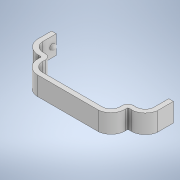
# Autodesk Inventor part: NEMA23_Shroud_Cover
Saved by Autodesk Inventor 2021 (Build 250183000, 183)
## iProperties
Created: 2021-04-01
Part Number: NEMA23_Shroud_Cover
Material: Generic
Document SubType Name: Modeling
Designer: Jorian Brusind
Density: 1 g/cm^3
Appearance: Default
Author: Jorian Brusind
Autodesk Inventor part; units mm, degrees
ref_plane "YZ Plane" through (0, 0, 0) normal (1, 0, 0) x (0, 1, 0)
ref_plane "XZ Plane" through (0, 0, 0) normal (0, 1, 0) x (-1, 0, 0)
ref_plane "XY Plane" through (0, 0, 0) normal (0, 0, 1) x (1, 0, 0)
sketch "Sketch1" plane through (0, 0, 0) normal (0, 1, 0) x (-1, 0, 0)
  arc A0 (-51.5269, -6.9638) -> (-48.7189, -4.3924) centre (-51.6928, -3.9638) ccw
  line L0 (-51.5269, -6.9638) -> (-53.0277, -6.9638)
  arc A1 (-53.0277, -6.9638) -> (-55.8647, -7.8466) centre (-53.0278, -11.9638) ccw
  arc A2 (-48.0059, -0.3912) -> (-48.7189, -2.9645) centre (-43.7189, -2.9645) ccw
  line L1 (-48.7189, -2.9645) -> (-48.7189, -4.3924)
  arc A3 (-44.3192, 1.9993) -> (-48.0059, -0.3912) centre (-43.7189, -2.9645) ccw
  arc A4 (-55.8647, -7.8466) -> (-57.9428, -11.046) centre (-53.0278, -11.9639) ccw
  arc A5 (-7.9592, -0.1638) -> (-12.0937, 1.9993) centre (-12.0765, -3.0006) ccw
  arc A6 (-7.0769, -2.9368) -> (-7.9592, -0.1638) centre (-12.0765, -3.0006) ccw
  arc A7 (-7.0717, -4.4481) -> (-4.4894, -7.4079) centre (-4.0718, -4.4371) ccw
  line L2 (-7.0717, -4.4481) -> (-7.0769, -2.9368)
  arc A8 (-0.4247, -8.1232) -> (-3.0701, -7.403) centre (-3.0107, -12.4029) ccw
  line L3 (-3.0701, -7.403) -> (-4.4894, -7.4079)
  arc A9 (2.1302, -12.0566) -> (-0.4247, -8.1232) centre (-2.8554, -12.4986) ccw
  line L4 (2.1302, -12.0566) -> (2.1302, -17.0566)
  line L5 (-57.9428, -11.046) -> (-57.9439, -17.046)
  line L6 (-57.9439, -17.046) -> (2.1302, -17.0566)
  line L7 (-44.3192, 1.9993) -> (-12.0937, 1.9993)
  arc A10 (-6.0769, -2.9289) -> (-7.1357, 0.4036) centre (-12.0765, -3.0006) ccw
  arc A11 (-7.1357, 0.4036) -> (-12.0953, 2.9993) centre (-12.0765, -3.0006) ccw
  line L8 (-12.0953, 2.9993) -> (-44.3767, 2.9993)
  arc A12 (-44.3767, 2.9993) -> (-48.8633, 0.1235) centre (-43.7189, -2.9645) ccw
  arc A13 (-48.8633, 0.1235) -> (-49.7189, -2.9645) centre (-43.7189, -2.9645) ccw
  line L9 (-49.7189, -2.9645) -> (-49.7189, -4.3135)
  arc A14 (-51.5573, -5.9638) -> (-49.7189, -4.3135) centre (-51.6928, -3.9638) ccw
  line L10 (-51.5573, -5.9638) -> (-53.0277, -5.9638)
  arc A15 (-53.0277, -5.9638) -> (-56.4321, -7.0231) centre (-53.0278, -11.9638) ccw
  arc A16 (-56.4321, -7.0231) -> (-58.9428, -10.9576) centre (-53.0278, -11.9639) ccw
  line L11 (-58.9428, -10.9576) -> (-58.9441, -18.0408)
  line L12 (3.1302, -18.0204) -> (3.1302, -12.0144)
  arc A17 (3.1302, -12.0144) -> (0.0768, -7.258) centre (-2.8554, -12.4986) ccw
  arc A18 (0.0768, -7.258) -> (-3.0776, -6.403) centre (-3.0107, -12.4029) ccw
  line L13 (-3.0776, -6.403) -> (-4.4139, -6.4076)
  arc A19 (-6.0717, -4.4446) -> (-4.4139, -6.4076) centre (-4.0718, -4.4371) ccw
  line L14 (-6.0717, -4.4446) -> (-6.0769, -2.9289)
  arc A20 (-4.577, -2.9177) -> (-5.9005, 1.2546) centre (-12.0765, -3.0006) ccw
  arc A21 (-5.9005, 1.2546) -> (-12.0976, 4.4993) centre (-12.0765, -3.0006) ccw
  line L15 (-12.0976, 4.4993) -> (-44.4545, 4.4993)
  arc A22 (-44.4545, 4.4993) -> (-50.1493, 0.8955) centre (-43.7189, -2.9645) ccw
  arc A23 (-50.1493, 0.8955) -> (-51.2189, -2.9645) centre (-43.7189, -2.9645) ccw
  line L16 (-51.2189, -2.9645) -> (-51.2189, -4.1372)
  arc A24 (-51.6249, -4.4638) -> (-51.2189, -4.1372) centre (-51.6928, -3.9638) ccw
  line L17 (-51.6249, -4.4638) -> (-53.0277, -4.4638)
  arc A25 (-53.0277, -4.4638) -> (-57.2832, -5.7879) centre (-53.0278, -11.9638) ccw
  arc A26 (-57.2832, -5.7879) -> (-60.4428, -10.8378) centre (-53.0278, -11.9639) ccw
  line L18 (-60.4428, -10.8378) -> (-60.4443, -19.5405)
  line L19 (4.6302, -19.5486) -> (4.6302, -11.9572)
  arc A27 (4.6302, -11.9572) -> (0.8291, -5.9601) centre (-2.8554, -12.4986) ccw
  arc A28 (0.8291, -5.9601) -> (-3.0882, -4.903) centre (-3.0107, -12.4029) ccw
  line L20 (-3.0882, -4.903) -> (-4.2426, -4.907)
  arc A29 (-4.5718, -4.4391) -> (-4.2426, -4.907) centre (-4.0718, -4.4371) ccw
  line L21 (-4.5718, -4.4391) -> (-4.577, -2.9177)
  line L22 (3.1302, -18.0204) -> (3.1302, -19.5486)
  line L23 (3.1302, -18.0204) -> (4.6584, -18.0204) construction
  line L24 (3.1302, -19.5486) -> (4.6302, -19.5486)
  line L25 (-58.9441, -18.0408) -> (-58.9441, -19.5405)
  line L26 (-58.9441, -19.5405) -> (-60.4443, -19.5405)
  line L27 (-58.9441, -19.5405) -> (-57.9439, -19.5405)
  line L28 (-57.9439, -19.5405) -> (-57.9439, -17.046)
  line L29 (3.1302, -19.5486) -> (2.1302, -19.5486)
  line L30 (2.1302, -19.5486) -> (2.1302, -17.0566)
  point P0 (0, 0)
  point P1 (0, 0)
  dimension "d5" = 5
  dimension "d6" = 6
  dimension "d8" = 3
  dimension "d11" = 1
  dimension "d12" = 1.5
  dimension "d13" = 90
  dimension "d16" = 1
  constraints: 62 end point, 60 point on circle, 30 centre point, 6 perpendicular, 4 horizontal, 1 vertical, 30 other
  measures "d5" distance of L4.start L4.end
  measures "d6" distance of L5.start L5.end
  measures "d8" radius of A7
  measures "d11" distance between parallel lines of L2 L14
  measures "d12" distance between parallel lines of L14 L21
  measures "d13" angle of L22 L23
  measures "d16" distance of L22.end L29.end
extrude "Extrusion2" add sketch "Sketch1" along normal blind 10 contours L0 A1 A4 L5 L28 L27 L25 L11 A16 A15 L10 A14 L9 A13 A12 L8 A11 A10 L14 A19 L13 A18 A17 L12 L22 L29 L30 L4 A9 A8 L3 A7 L2 A6 A5 L7 A3 A2 L1 A0 | L26 L18 A26 A25 L17 A24 L16 A23 A22 L15 A21 A20 L21 A29 L20 A28 A27 L19 L24 L22 L12 A17 A18 L13 A19 L14 A10 A11 L8 A12 A13 L9 A14 L10 A15 A16 L11 L25
sketch "Sketch2" plane through (-2.1302, 0, -12.0566) normal (1, 0, 0) x (0, 0, -1)
  line L0 (7.492, 0) -> (7.492, 10) projected
  line L1 (7.492, 5) -> (5.492, 5)
  arc A0 (6.992, 5) -> (3.992, 5) centre (5.492, 5) ccw
  line L2 (5.492, 5) -> (3.992, 5)
  point P0 (-12.0566, 0)
  dimension "d19" = 2
  dimension "d21" = 1.5
  constraints: 4 end point, 2 horizontal, 2 point on circle, 1 centre point, 1 coincident, 1 midpoint, 1 point on line
  measures "d19" distance of L1.start L1.end
  measures "d21" radius of A0
revolve "Revolution1" add sketch "Sketch2" angle 360 about axis through (-2.1302, 5, -19.5486) along (0, 0, 1)
sketch "Sketch3" plane through (57.9439, 0, -19.5405) normal (-1, 0, 0) x (0, 0, 1)
  line L0 (0, 0) -> (0, 10) projected
  line L1 (0, 5) -> (2, 5)
  arc A0 (3.5, 5) -> (0.5, 5) centre (2, 5) ccw
  line L2 (2, 5) -> (3.5, 5)
  point P0 (19.5405, 0)
  point P1 (2, 5)
  dimension "d23" = 2
  dimension "d24" = 1.5
  constraints: 4 end point, 2 horizontal, 2 point on circle, 1 centre point, 1 coincident, 1 midpoint, 1 point on line
  measures "d23" distance of L1.start L1.end
  measures "d24" radius of A0
revolve "Revolution2" add sketch "Sketch3" angle 360 about axis through (57.9439, 5, -19.5405) along (0, 0, 1)
body "Solid2"
